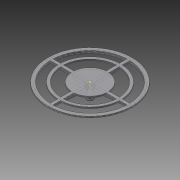
# Autodesk Inventor part: rotating platform
Saved by Autodesk Inventor 2015 (Build 190159000, 159)
## iProperties
Created: 2019-01-11
Part Number: rotating platform
Material: Generic
Document SubType Name: Modeling
Designer: Toby
Density: 1 g/cm^3
Appearance: Default
Author: Toby
Autodesk Inventor part; units mm, degrees
ref_plane "YZ Plane" through (0, 0, 0) normal (1, 0, 0) x (0, 1, 0)
ref_plane "XZ Plane" through (0, 0, 0) normal (0, 1, 0) x (-1, 0, 0)
ref_plane "XY Plane" through (0, 0, 0) normal (0, 0, 1) x (1, 0, 0)
sketch "Sketch1" plane through (0, 0, 0) normal (0, 0, 1) x (1, 0, 0)
  circle A0 centre (0, 0) radius 2.6
  circle A1 centre (0, 0) radius 5
  dimension "d0" = 5.2
  dimension "d1" = 10
  constraints: 2 centre point, 2 coincident
  measures "d0" diameter of A0
  measures "d1" diameter of A1
extrude "Extrusion1" add sketch "Sketch1" along normal blind 20
sketch "Sketch2" plane through (0, 0, 20) normal (0, 0, 1) x (1, 0, 0)
  circle A0 centre (0, 0) radius 25
  dimension "d4" = 50
  constraints: 1 centre point, 1 coincident
  measures "d4" diameter of A0
extrude "Extrusion2" add sketch "Sketch2" against normal blind 2
sketch "Sketch3" plane through (0, 0, 18) normal (0, 0, -1) x (-1, 0, 0)
  line L0 (2, 22) -> (-2, 22)
  line L1 (-2, 22) -> (-2, 2.7)
  line L2 (-2, 2.7) -> (2, 2.7)
  line L3 (2, 2.7) -> (2, 22)
  line L4 (2, -3.131) -> (-2, -3.131)
  line L5 (-2, -3.131) -> (-2, -22)
  line L6 (-2, -22) -> (2, -22)
  line L7 (2, -22) -> (2, -3.131)
  line L8 (3.392, 2) -> (22, 2)
  line L9 (22, 2) -> (22, -2)
  line L10 (22, -2) -> (3.392, -2)
  line L11 (3.392, -2) -> (3.392, 2)
  line L12 (-3.6849, 2) -> (-22, 2)
  line L13 (-22, 2) -> (-22, -2)
  line L14 (-22, -2) -> (-3.6849, -2)
  line L15 (-3.6849, -2) -> (-3.6849, 2)
  point P0 (0, 0)
  dimension "d7" = 2
  dimension "d8" = 2
  dimension "d9" = 2
  dimension "d10" = 2
  dimension "d11" = 22
  dimension "d12" = 22
  dimension "d13" = 22
  dimension "d14" = 22
  dimension "d15" = 2.7
  constraints: 32 end point, 8 parallel, 4 horizontal, 4 perpendicular, 4 point on line
  measures "d7" distance from line of point (0, 0) L3
  measures "d8" distance from line of point (0, 0) L1
  measures "d9" distance from line of point (0, 0) L8
  measures "d10" distance from line of point (0, 0) L10
  measures "d11" distance from line of point (0, 0) L9
  measures "d12" distance from line of point (0, 0) L0
  measures "d13" distance from line of point (0, 0) L6
  measures "d14" distance from line of point (0, 0) L13
  measures "d15" distance from line of point (0, 0) L2
extrude "Extrusion3" add sketch "Sketch3" along normal blind 1.5
chamfer "Chamfer1" distance 1.5 angle 45 1 edges at (22, 0, 18)
chamfer "Chamfer2" distance 1.5 angle 45 1 edges at (0, -22, 18)
chamfer "Chamfer3" distance 1.5 angle 45 1 edges at (-22, 0, 18)
chamfer "Chamfer4" distance 1.5 angle 45 1 edges at (0, 22, 18)
sketch "Sketch4" plane through (0, 0, 0) normal (1, 0, 0) x (0, 1, 0)
  line L0 (-5, 0) -> (5, 0) projected
  point P0 (0, 0)
  point P1 (0, 10)
  dimension "d30" = 10
  measures "d30" distance from line of L0 point (0, 10)
hole "Hole1" at (0, 0, 10) direction (-1, 0, 0) diameter 3 depth 8 tip angle 118
sketch "Sketch5" plane through (0, 0, 20) normal (0, 0, 1) x (1, 0, 0)
  point P0 (0, 0)
sketch "Sketch6" plane through (0, 0, 20) normal (0, 0, 1) x (1, 0, 0)
  line L0 (-2, -4.5826) -> (2, -4.5826)
  line L1 (2, -4.5826) -> (2, -59.5826)
  line L2 (2, -59.5826) -> (-2, -59.5826)
  line L3 (-2, -59.5826) -> (-2, -4.5826)
  line L4 (-2, 4.5826) -> (2, 4.5826)
  line L5 (2, 4.5826) -> (2, 59.5826)
  line L6 (2, 59.5826) -> (-2, 59.5826)
  line L7 (-2, 59.5826) -> (-2, 4.5826)
  line L8 (4.5826, -2) -> (59.5826, -2)
  line L9 (59.5826, -2) -> (59.5826, 2)
  line L10 (59.5826, 2) -> (4.5826, 2)
  line L11 (4.5826, 2) -> (4.5826, -2)
  arc A0 (-4.5826, 2) -> (-4.5826, -2) centre (0, 0) ccw projected
  line L12 (-4.5826, -2) -> (-59.5826, -2)
  line L13 (-59.5826, -2) -> (-59.5826, 2)
  line L14 (-59.5826, 2) -> (-4.5826, 2)
  line L15 (-4.5826, 2) -> (-4.5826, -2)
  dimension "d38" = 55
  dimension "d39" = 55
  dimension "d40" = 55
  dimension "d41" = 55
  constraints: 32 end point, 8 parallel, 4 horizontal, 4 perpendicular, 3 point on line, 1 point on circle
  measures "d38" distance of L0.end L1.end
  measures "d39" distance of L5.end L4.end
  measures "d40" distance of L10.end L9.end
  measures "d41" distance of L13.end L14.end
extrude "Extrusion4" add sketch "Sketch6" against normal blind 2
chamfer "Chamfer5" distance 1.5 angle 45 4 edges at (0, -59.5826, 18) (59.5826, 0, 18) (0, 59.5826, 18) (-59.5826, 0, 18)
sketch "Sketch7" plane through (0, 0, 18) normal (0, 0, -1) x (-1, 0, 0)
  circle A0 centre (0, 0) radius 60
  circle A1 centre (0, 0) radius 55
  dimension "d47" = 5
  dimension "d48" = 120
  constraints: 2 centre point, 2 coincident
  measures "d47" radial gap between concentric circles of A0 A1
  measures "d48" diameter of A0
extrude "Extrusion5" add sketch "Sketch7" against normal blind 2
sketch "Sketch8" plane through (0, 0, 18) normal (0, 0, -1) x (-1, 0, 0)
  circle A0 centre (0, 0) radius 60 projected
  line L0 (-2, -4.5826) -> (2, -4.5826)
  line L1 (2, -4.5826) -> (2, -59.9667)
  line L2 (2, -59.9667) -> (-2, -59.9667)
  line L3 (-2, -59.9667) -> (-2, -4.5826)
  line L4 (2, -54.9636) -> (2, -24.9199) projected
  line L5 (-2, 4.5826) -> (2, 4.5826)
  line L6 (2, 4.5826) -> (2, 59.9667)
  line L7 (2, 59.9667) -> (-2, 59.9667)
  line L8 (-2, 59.9667) -> (-2, 4.5826)
  line L9 (4.5826, -2) -> (59.9667, -2)
  line L10 (59.9667, -2) -> (59.9667, 2)
  line L11 (59.9667, 2) -> (4.5826, 2)
  line L12 (4.5826, 2) -> (4.5826, -2)
  arc A1 (-4.5826, 2) -> (-4.5826, -2) centre (0, 0) ccw projected
  line L13 (-4.5826, -2) -> (-59.9667, -2)
  line L14 (-59.9667, -2) -> (-59.9667, 2)
  line L15 (-59.9667, 2) -> (-4.5826, 2)
  line L16 (-4.5826, 2) -> (-4.5826, -2)
  constraints: 32 end point, 8 parallel, 5 point on circle, 4 horizontal, 4 perpendicular, 2 point on line, 1 collinear
extrude "Extrusion6" add sketch "Sketch8" along normal blind 5 contours L10 L9 L12 L11 | L6 L5 L8 L7 | L2 L3 L0 L1 | L15 A1 L13 L14 | L16 A1
chamfer "Chamfer6" distance 55 distance2 5 1 edges at (0, -59.9667, 13) measured on face at (0, -59.4667, 13)
chamfer "Chamfer7" distance 55 distance2 5 1 edges at (0, 59.9667, 13) measured on face at (0, 59.4667, 13)
chamfer "Chamfer8" distance 55 distance2 5 1 edges at (59.9667, 0, 13) measured on face at (59.4667, 0, 13)
chamfer "Chamfer9" distance 55 distance2 5 1 edges at (-59.9667, 0, 13) measured on face at (-59.4667, 0, 13)
sketch "Sketch9" plane through (0, 0, 20) normal (0, 0, 1) x (1, 0, 0)
  circle A0 centre (0, 0) radius 40
  circle A1 centre (0, 0) radius 44
  dimension "d65" = 80
  dimension "d66" = 88
  constraints: 2 centre point, 2 coincident
  measures "d65" diameter of A0
  measures "d66" diameter of A1
extrude "Extrusion7" add sketch "Sketch9" against normal blind 2
sketch "Sketch10" plane through (0, 0, 18) normal (0, 0, -1) x (-1, 0, 0)
  circle A0 centre (0, 0) radius 2.6 projected
  circle A1 centre (0, 0) radius 55
  circle A2 centre (0, 0) radius 57
  dimension "d69" = 110
  dimension "d70" = 2
  constraints: 2 centre point, 2 coincident
  measures "d69" diameter of A1
  measures "d70" radial gap between concentric circles of A1 A2
extrude "Extrusion8" add sketch "Sketch10" along normal blind 2 contours A2
body "Solid1"
